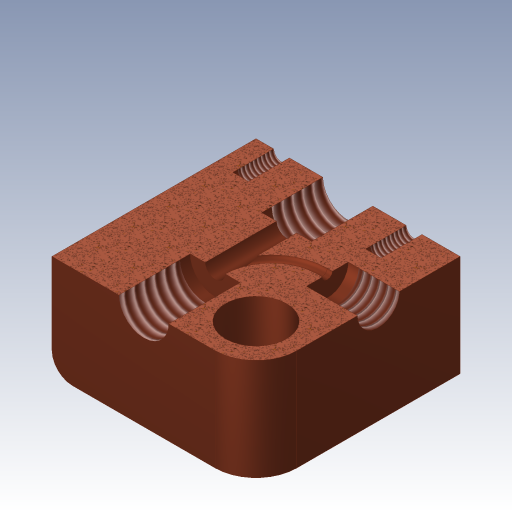
# Autodesk Inventor part: BT001_huenin20_23
Saved by Autodesk Inventor 2023.3 (Build 273359000, 359)
## iProperties
Company: HTBLA Kaindorf
RuleStatus: InUse
AfterDocNew0: iProperties-Editor_aufrufen
Created: 2023-05-23
Part Number: BT001_huenin20_23
Project: Fiberprinter-Hotend
Material: Kupfer
Description: Heizblock
Document SubType Name: Modeling
Designer: huenin20
Density: 8.94 g/cm^3
Appearance: Kupfer - satiniert
Mass: 61.3246 g
Surface Area: 31.335 cm^2
Volume: 6.85958 cm^3
Author: nicob
Keywords: 2023
Autodesk Inventor part; units mm, degrees
ref_plane "YZ Plane" through (0, 0, 0) normal (1, 0, 0) x (0, 1, 0)
ref_plane "XZ Plane" through (0, 0, 0) normal (0, 1, 0) x (-1, 0, 0)
ref_plane "XY Plane" through (0, 0, 0) normal (0, 0, 1) x (1, 0, 0)
sketch "Skizze3" plane through (0, 0, 0) normal (0, 0, 1) x (1, 0, 0)
  line L0 (0, 0) -> (-20, 0)
  line L1 (-20, 0) -> (-20, 20)
  line L2 (-20, 20) -> (0, 20)
  line L3 (0, 20) -> (0, 0)
  line L4 (-20, 9) -> (0, 9)
  circle A0 centre (-4.5, 15.5) radius 3
  arc A1 (-12, 14.5) -> (-7, 9.5) centre (-7, 14.5) ccw
  line L5 (-12, 14.5) -> (-12, 20)
  dimension "d4" = 20
  dimension "d5" = 20
  dimension "d68" = 9
  dimension "d115" = 6
  dimension "d116" = 4.5
  dimension "d117" = 4.5
  dimension "d118" = 1
  dimension "d119" = 7
  dimension "d120" = 8
  dimension "d121" = 5
  constraints: 12 end point, 3 perpendicular, 3 point on line, 2 centre point, 2 parallel, 2 point on circle, 1 horizontal, 1 tangent
  measures "d4" distance of L1.end L2.end
  measures "d5" distance of L0.end L1.end
  measures "d68" distance from line of L0 L4.start
  measures "d115" diameter of A0
  measures "d116" distance from line of L2 A0.centre
  measures "d117" distance from line of L3 A0.centre
  measures "d118" diameter of A1.end L4
  measures "d119" distance from line of L3 A1.end
  measures "d120" distance between parallel lines of L1 L5
  measures "d121" radius of A1
extrude "Extrusion3" add sketch "Skizze3" along normal mid plane 20
sketch "Skizze12" plane through (-20, 0, 10) normal (-1, 0, 0) x (0, 0, 1)
  point P0 (-10, 0)
  point P1 (-10, 9)
hole "Bohrung4" at (-20, 9, 0) direction (1, 0, 0) diameter 4.917 depth 6
hole "Bohrung5" at (-20, 9, 0) direction (1, 0, 0) diameter 2 end through all
sketch "Skizze13" plane through (0, 0, 10) normal (1, 0, 0) x (0, 0, -1)
  point P0 (10, 0)
  point P1 (10, 9)
hole "Bohrung7" at (0, 9, 0) direction (-1, 0, 0) diameter 4.917 depth 7
sketch "Skizze14" plane through (-20, 20, 10) normal (0, 1, 0) x (1, 0, 0)
  circle A0 centre (8, 10) radius 0.5
  point P0 (20, 10)
  point P1 (8, 10)
  dimension "d129" = 1
  constraints: 1 centre point, 1 coincident
  measures "d129" diameter of A0
hole "Bohrung8" at (-12, 20, 0) direction (0, -1, 0) diameter 4.134 depth 5
sweep "Sweeping3" cut profiles "Skizze14" path "Skizze3" path curves L5 A1
fillet "Rundung3" radius 4 1 edges at (0, 20, 0)
sketch "Skizze18" plane through (-20, 0, 10) normal (-1, 0, 0) x (0, 0, 1)
  line L0 (-20, 0) -> (-20, 20) projected
  line L1 (-20, 20) -> (0, 20) projected
  line L2 (0, 0) -> (0, 16) projected
  line L3 (0, 9) -> (-20, 9) construction
  line L4 (-20, 16) -> (-20, 0) projected
  point P0 (-10, 0)
  point P1 (-16.5, 15.5)
  point P2 (-3.5, 15.5)
  point P3 (-10, 15.5)
  point P4 (-16.5, 2.5)
  point P5 (-3.5, 2.5)
  point P6 (-10, 2.5)
  point P7 (-10, 9)
  dimension "d192" = 13
  dimension "d194" = 4.5
  dimension "d210" = 6.5
  dimension "d229" = 11
  constraints: 3 symmetric about line, 2 end point, 2 horizontal alignment, 2 point on line, 1 midpoint, 1 perpendicular, 1 vertical alignment
  measures "d192" distance of point (-16.5, 15.5) point (-3.5, 15.5)
  measures "d194" distance from line of L1 point (-3.5, 15.5)
  measures "d210" distance of point (-16.5, 15.5) point (-10, 15.5)
  measures "d229" distance between parallel lines of L1 L3
hole "Bohrung13" at (-20, 15.5, 6.5) at (-20, 15.5, -6.5) at (-20, 2.5, -6.5) at (-20, 2.5, 6.5) direction (1, 0, 0) diameter 3.5 depth 3
hole "Bohrung16" at (-20, 15.5, 0) at (-20, 2.5, 0) direction (1, 0, 0) diameter 1.567 depth 4
fillet "Rundung4" radius 2 2 edges at (-10, 0, 10) (-10, 0, -10)
equation "\"Heizpatronen_durchmesser\" = 6"
